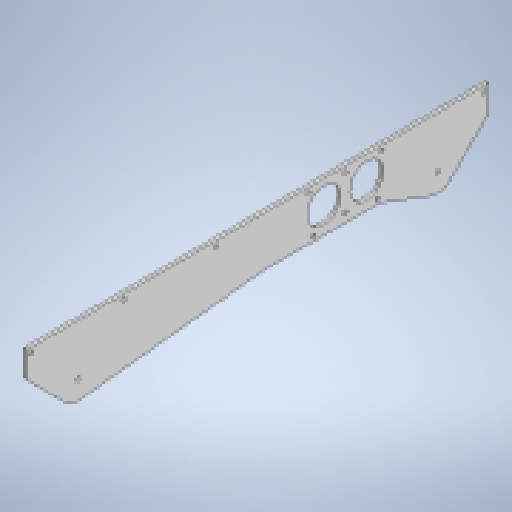
# Autodesk Inventor part: insideChassiPlate
Saved by Autodesk Inventor 2023 (Build 270158000, 158)
## iProperties
Created: 2022-09-05
Part Number: insideChassiPlate
Material: Generic
Document SubType Name: Modeling
Designer: deli
Density: 1 g/cm^3
Appearance: Default
Author: deli
Autodesk Inventor part; units mm, degrees
ref_plane "YZ Plane" through (0, 0, 0) normal (1, 0, 0) x (0, 1, 0)
ref_plane "XZ Plane" through (0, 0, 0) normal (0, 1, 0) x (-1, 0, 0)
ref_plane "XY Plane" through (0, 0, 0) normal (0, 0, 1) x (1, 0, 0)
sketch "Sketch1" plane through (0, 0, 0) normal (1, 0, 0) x (0, 1, 0)
  arc A0 (67.9768, 91.2638) -> (62.7594, 76.28) centre (80.627, 78.4587) ccw projected
  line L0 (62.7594, 76.28) -> (82.627, -86.6583) projected
  line L1 (82.627, -86.6583) -> (82.627, -221.3779) projected
  line L2 (82.627, -221.3779) -> (64.0942, -264.4233) projected
  arc A1 (64.0942, -264.4233) -> (67.9768, -284.3465) centre (80.627, -271.5413) ccw projected
  line L3 (67.9768, -284.3465) -> (105.627, -321.5413) projected
  line L4 (105.627, -321.5413) -> (130.627, -321.5413) projected
  line L5 (130.627, -321.5413) -> (130.627, 128.4587) projected
  line L6 (130.627, 128.4587) -> (105.627, 128.4587) projected
  line L7 (105.627, 128.4587) -> (67.9768, 91.2638) projected
  circle A2 centre (80.627, -271.5413) radius 2 projected
  circle A3 centre (110.627, -161.0021) radius 7 projected
  circle A4 centre (110.627, -203.8739) radius 7 projected
  circle A5 centre (80.627, 78.4587) radius 2 projected
  circle A6 centre (110.627, -161.0021) radius 16.5
  circle A7 centre (110.627, -203.8739) radius 16.5
  circle A8 centre (122.627, -220.4946) radius 2 projected
  circle A9 centre (122.627, -144.3813) radius 2 projected
  circle A10 centre (121.4207, -182.438) radius 2 projected
  circle A11 centre (99.8334, -182.438) radius 2 projected
  circle A12 centre (90.627, -156.5021) radius 2 projected
  circle A13 centre (90.627, -208.3739) radius 2 projected
  circle A14 centre (125.627, -55.1125) radius 2 projected
  circle A15 centre (125.627, -316.5413) radius 2 projected
  circle A16 centre (125.627, 123.4587) radius 2 projected
  circle A17 centre (125.627, 34.1731) radius 2 projected
  point P0 (0, 0)
  dimension "d0" = 33
  dimension "d1" = 33
  constraints: 2 centre point, 2 coincident
  measures "d0" diameter of A6
  measures "d1" diameter of A7
extrude "Extrusion1" add sketch "Sketch1" along normal blind 3.175 contours L7 L6 L5 L4 L3 A1 L2 L1 L0 A0
equation "\"d1\" = d0"
body "Solid1"
